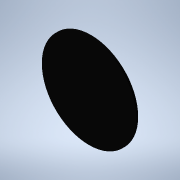
# Autodesk Inventor part: EGC-80-TB-KF__(CUP)
Saved by Autodesk Inventor 2021 (Build 250183000, 183)
## iProperties
Created: 2026-04-25
Part Number: EGC-80-TB-KF__(CUP)
Material: Generic
Catalog Web Link: www.3dfindit.com
Description: EGC-TB-CUPS-Cups
Vendor: FESTO
Document SubType Name: Modeling
Designer: psAdmin
Manufacturer: FESTO
Mass: 1.80956 g
Surface Area: 37.6991 cm^2
Volume: 1.80956 cm^3
Density: 1 g/cm^3
Appearance: PSOLRGB-80-80-80
Category: PARTsolutions
Company: FESTO
Title: EGC-80-TB-KF__(CUP)
Author: Cadenas PARTsolutions
Comments: Cups
PSOL_IDENT_0: {$CADENAS_DATA/23d-libs/festo/parts/e/egc/parts/egc_tb_cup.prj},183 {VTYP=3D},{NB=EGC-80-TB-KF__(CUP
PSOL_IDENT_1: )},{LINA=EGC-80-TB-KF__(CUP)},{NN=EGC-TB-CUPS},{DATE=08.09.2025 12:26:32},{GEOMDATE=02.09.2015 14:27
PSOL_IDENT_2: :23},{VERSION=},{LINEID=30},{WBVAR=},{WBNUMERIC=}  {NB=EGC-80-TB-KF__(CUP)},{LINA=EGC-80-TB-KF__(CUP
PSOL_IDENT_3: )},{KT=DUMMY},{TYP=EGC-80-TB-KF},{VERS=3.000},{SIZE=80.000},{D=48.000},{B=1.000}
NB: EGC-80-TB-KF__(CUP)
NN: EGC-TB-CUPS
NT: Cups
NBSYN: $TYP.__(CUP)
LINA: EGC-80-TB-KF__(CUP)
CATALOG: Festo
TYP: EGC-80-TB-KF
VERS: 3
SIZE: 80
D: 48
B: 1
SUPPLIER: FESTO
ARTICLENO: EGC-80-TB-KF__(CUP)
BOMINFO: EGC-80-TB-KF__(CUP)
CREATOR: CADENAS GmbH
Autodesk Inventor part; units mm, degrees
sketch "Sketch_1" plane through (0, 0, 0) normal (0, 0, 1) x (1, 0, 0)
  circle A0 centre (0, 0) radius 24
  constraints: 1 centre point
extrude "Extrusion1" add sketch "Sketch_1" against normal blind 1
ref_plane "CUP_XY" through (0, 0, 0) normal (0, 0, 1) x (1, 0, 0)
ref_plane "CUP_YZ" through (0, 0, 0) normal (1, 0, 0) x (0, 1, 0)
ref_plane "CUP_ZX" through (0, 0, 0) normal (0, 1, 0) x (0, 0, 1)
body "Solid1"
